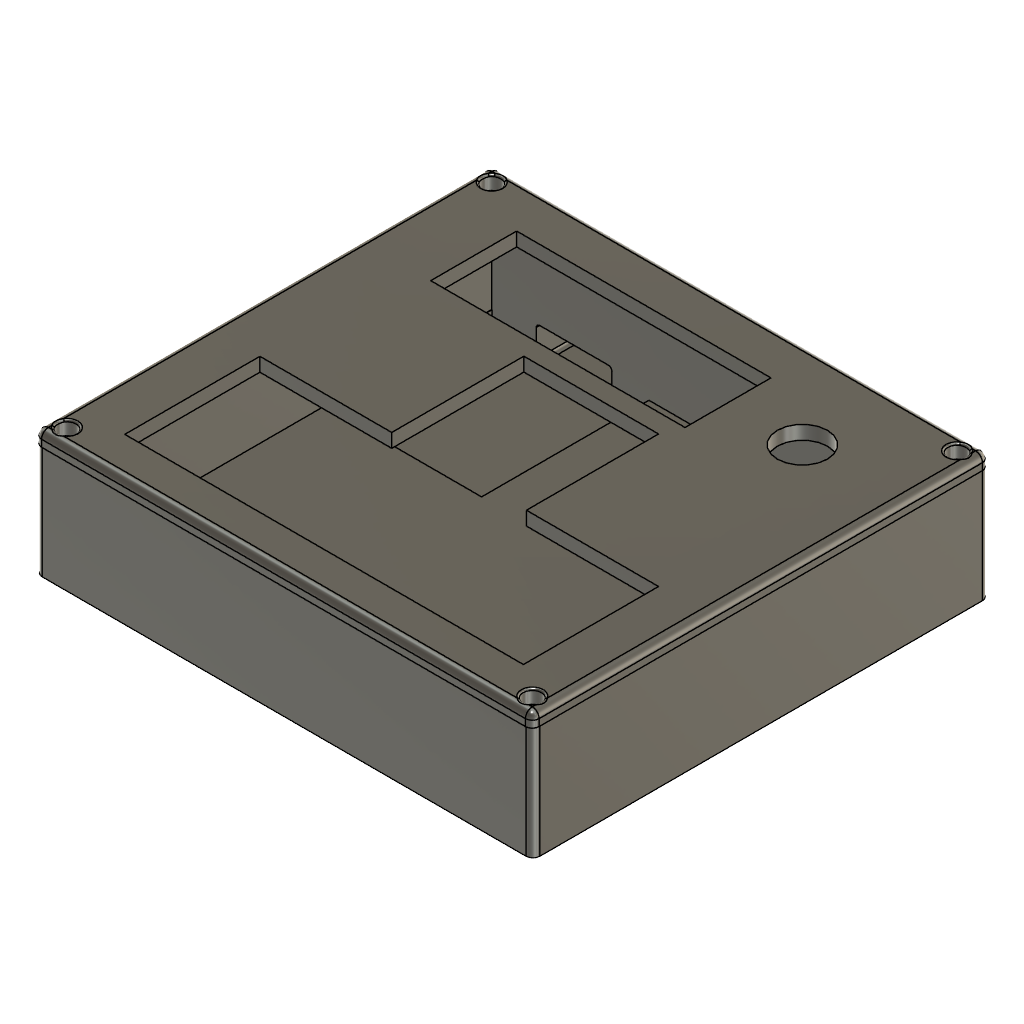
full render of de macropad (Autodesk Fusion 360 archive; units mm, degrees)
design "hackpad"
Autodesk Fusion 360 part; units mm, degrees
sketch "Sketch1" plane through (0, 0, 0) normal (0, 0, 1) x (1, 0, 0)
  line L0 (-90.4808, 59.85) -> (-28.0808, 59.85)
  line L1 (-28.0808, 59.85) -> (-28.0808, 3.45)
  line L2 (-28.0808, 3.45) -> (-90.4808, 3.45)
  line L3 (-90.4808, 3.45) -> (-90.4808, 59.85)
  dimension "d1" = 62.4
  dimension "d2" = 56.4
  constraint horizontal L0
  constraint vertical L1
  constraint horizontal L2
  constraint vertical L3
  measures "d1" distance of L0.start L0.end
  measures "d2" distance of L0.start L2.end
extrude "Extrude1" add sketch "Sketch1" along normal blind 11.4 makes body 1
shell "Shell1" thickness 5 outward yes removed faces 1 at (-69.6808, 41.05, 11.4) on bodies 1
ref_plane "WorkPlane1" through (-59.2808, 31.65, 11.4) normal (0, 0, 1) x (1, 0, 0)
sketch "Sketch2" plane through (0, 0, 11.4) normal (0, 0, 1) x (1, 0, 0)
  line L0 (-95.48, 64.8499) -> (-23.0806, 64.8499)
  line L1 (-23.0806, 64.8499) -> (-23.0806, -1.6501)
  line L2 (-23.0806, -1.6501) -> (-95.48, -1.6501)
  line L3 (-95.48, -1.6501) -> (-95.48, 64.8499)
  line L4 (-88.0462, 23.6829) -> (-30.0462, 23.6829)
  line L5 (-30.0462, 23.6829) -> (-30.0462, 4.0249)
  line L6 (-30.0462, 4.0249) -> (-88.0462, 4.0249)
  line L7 (-88.0462, 4.0249) -> (-88.0462, 23.6829)
  line L8 (-68.8631, 23.6829) -> (-49.2669, 23.6829)
  line L9 (-49.2669, 23.6829) -> (-49.2669, 42.9032)
  line L10 (-49.2669, 42.9032) -> (-68.8631, 42.9032)
  line L11 (-68.8631, 42.9032) -> (-68.8631, 23.6829)
  circle A0 centre (-37.446, 52.0157) radius 3.64
  line L12 (-85.1542, 58.1457) -> (-48.1542, 58.1457)
  line L13 (-48.1542, 58.1457) -> (-48.1542, 45.6457)
  line L14 (-48.1542, 45.6457) -> (-85.1542, 45.6457)
  line L15 (-85.1542, 45.6457) -> (-85.1542, 58.1457)
  dimension "d7" = 7.28
  dimension "d10" = 37
  dimension "d11" = 12.5
  dimension "d38" = 66.5
  constraint horizontal L0
  constraint vertical L1
  constraint horizontal L2
  constraint vertical L3
  constraint horizontal L4
  constraint vertical L5
  constraint horizontal L6
  constraint vertical L7
  constraint horizontal L8
  constraint vertical L9
  constraint horizontal L10
  constraint vertical L11
  constraint coincident L4 L8.start
  constraint horizontal L12
  constraint vertical L13
  constraint horizontal L14
  constraint vertical L15
  measures "d7" diameter of A0
  measures "d10" distance of L12.start L12.end
  measures "d11" distance of L12.start L14.end
  measures "d38" distance of L0.end L1.end
extrude "Extrude2" add sketch "Sketch2" along normal blind 2 separate body makes body 2
sketch "Sketch3" plane through (0, 0, 13.4) normal (0, 0, 1) x (-1, 0, 0)
  line L0 (49.2669, -42.9032) -> (49.2669, -23.6829)
  line L1 (49.2669, -23.6829) -> (30.0462, -23.6829)
  line L2 (30.0462, -23.6829) -> (30.0462, -4.0249)
  line L3 (30.0462, -4.0249) -> (88.0462, -4.0249)
  line L4 (88.0462, -4.0249) -> (88.0462, -23.6829)
  line L5 (88.0462, -23.6829) -> (68.8631, -23.6829)
  line L6 (68.8631, -23.6829) -> (68.8631, -42.9032)
  line L7 (68.8631, -42.9032) -> (49.2669, -42.9032)
  line L8 (48.1542, -45.6457) -> (85.1542, -45.6457)
  line L9 (85.1542, -45.6457) -> (85.1542, -58.1457)
  line L10 (85.1542, -58.1457) -> (48.1542, -58.1457)
  line L11 (48.1542, -58.1457) -> (48.1542, -45.6457)
  line L12 (95.48, 1.6501) -> (23.0806, 1.6501)
  line L13 (23.0806, 1.6501) -> (23.0806, -64.8499)
  line L14 (23.0806, -64.8499) -> (95.48, -64.8499)
  line L15 (95.48, -64.8499) -> (95.48, 1.6501)
  circle A0 centre (37.446, -52.0157) radius 3.64
sketch "Sketch4" plane through (0, 64.85, 0) normal (0, 1, 0) x (-1, 0, 0)
  line L0 (23.0808, -5) -> (95.4808, -5)
  line L1 (95.4808, -5) -> (95.4808, 11.4)
  line L2 (95.4808, 11.4) -> (23.0808, 11.4)
  line L3 (23.0808, 11.4) -> (23.0808, -5)
  line L4 (73, -3.5) -> (84, -3.5)
  line L5 (84, -3.5) -> (84, 1.4757)
  line L6 (84, 1.4757) -> (73, 1.4757)
  line L7 (73, 1.4757) -> (73, -3.5)
  constraint horizontal L4
  constraint vertical L5
  constraint horizontal L6
  constraint vertical L7
extrude "Extrude4" cut sketch "Sketch4" against normal blind 5 contours L4 L5 L6 L7 bodies 1
fillet "Fillet1" radius 1 4 edges at (-59.2803, -1.6501, 13.4) (-23.0806, 31.5999, 13.4) (-95.48, 31.5999, 13.4) (-59.2803, 64.8499, 13.4) on bodies 2
fillet "Fillet3" radius 1 12 edges at (-95.4808, -1.55, 3.2) (-23.0808, -1.55, 3.2) (-23.0808, 64.85, 3.2) (-95.4808, 64.85, 3.2) (-23.0806, -1.6501, 11.9) (-23.3735, -1.3572, 13.1071) (-95.48, -1.6501, 11.9) (-95.1871, -1.3572, 13.1071) (-23.3735, 64.557, 13.1071) (-23.0806, 64.8499, 11.9) (-95.1871, 64.557, 13.1071) (-95.48, 64.8499, 11.9) on bodies 1 2
fillet "Fillet3" radius 0.5 4 edges at (-73, 62.35, -3.5) (-73, 62.35, 1.4757) (-84, 62.35, -3.5) (-84, 62.35, 1.4757) on bodies 1 2
sketch "Sketch8" plane through (0, 0, 13.4) normal (0, 0, 1) x (-1, 0, 0)
  line L0 (94.48, 0.6501) -> (94.48, -63.8499)
  line L1 (94.48, -63.8499) -> (24.0806, -63.8499)
  circle A0 centre (93.13, -62.4999) radius 1.35
  line L2 (24.0806, 0.6501) -> (94.48, 0.6501)
  circle A1 centre (93.13, -0.6999) radius 1.35
  line L3 (24.0806, -63.8499) -> (24.0806, 0.6501)
  circle A2 centre (25.4306, -62.4999) radius 1.35
  circle A3 centre (25.4306, -0.6999) radius 1.35
  dimension "d39" = 1.35
  dimension "d40" = 1.35
  dimension "d41" = 1.35
  dimension "d42" = 1.35
  constraint tangent L0 A0
  constraint tangent L1 A0
  constraint tangent L0 A1
  constraint tangent L2 A1
  constraint tangent L1 A2
  constraint tangent L3 A2
  constraint tangent L3 A3
  constraint tangent L2 A3
  measures "d39" radius of A0
  measures "d40" radius of A1
  measures "d41" radius of A2
  measures "d42" radius of A3
extrude "Extrude6" cut sketch "Sketch8" against normal blind 7 contours A1 | A0 | A3 | A2 bodies 1 2
sketch "Sketch7" plane through (0, 0, 0) normal (0, 0, 1) x (-1, 0, 0)
  line L0 (28.0808, -59.85) -> (73, -59.85)
  line L1 (90.4808, -59.85) -> (90.4808, -3.45)
  line L2 (90.4808, -3.45) -> (28.0808, -3.45)
  line L3 (28.0808, -3.45) -> (28.0808, -59.85)
  line L4 (28.0808, -59.85) -> (90.4808, -59.85)
  line L5 (90.4808, -59.85) -> (90.4808, -3.45)
  line L6 (90.4808, -3.45) -> (28.0808, -3.45)
  line L7 (28.0808, -3.45) -> (28.0808, -59.85)
  line L8 (73, -59.85) -> (84, -59.85)
  line L9 (84, -59.85) -> (90.4808, -59.85)
  constraint horizontal L4
  constraint vertical L5
  constraint horizontal L6
  constraint vertical L7
  constraint coincident L1.end L2.start
  constraint coincident L0.start L3.end
fillet "Fillet4" radius 0.25 8 edges at (-92.1754, 61.5453, 13.4) (-94.0846, 63.4545, 13.4) (-92.1754, 1.6545, 13.4) (-94.0846, -0.2547, 13.4) (-26.3852, 1.6545, 13.4) (-24.476, -0.2547, 13.4) (-26.3852, 61.5453, 13.4) (-24.476, 63.4545, 13.4) on bodies 2
sketch "Sketch9" plane through (0, 0, 0) normal (0, 0, 1) x (-1, 0, 0)
  line L0 (28.0808, -59.85) -> (73, -59.85)
  line L1 (90.4808, -59.85) -> (90.4808, -3.45)
  line L2 (90.4808, -3.45) -> (28.0808, -3.45)
  line L3 (28.0808, -3.45) -> (28.0808, -59.85)
  line L4 (90.429, -59.85) -> (67.6096, -59.85)
  line L5 (67.6096, -59.85) -> (67.6096, -35.5043)
  line L6 (67.6096, -35.5043) -> (90.429, -35.5043)
  line L7 (90.429, -35.5043) -> (90.429, -59.85)
  line L8 (73, -59.85) -> (84, -59.85)
  line L9 (84, -59.85) -> (90.4808, -59.85)
  constraint horizontal L4
  constraint vertical L5
  constraint horizontal L6
  constraint vertical L7
  constraint coincident L0 L4.start
extrude "Extrude7" cut sketch "Sketch9" against normal blind 3.4 contours L0 L4 L5 L6 L7 L8 L9 bodies 1
